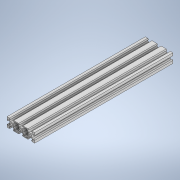
# Autodesk Inventor part: V-SLOT_2060
Saved by Autodesk Inventor 2021 (Build 250183000, 183)
## iProperties
Created: 2022-05-21
Part Number: V-SLOT_2060
Material: Genérico
Document SubType Name: Modeling
Designer: 79449
Density: 1 g/cm^3
Appearance: Valor por defecto
Author: 79449
Autodesk Inventor part; units mm, degrees
ref_plane "YZ Plane" through (0, 0, 0) normal (1, 0, 0) x (0, 1, 0)
ref_plane "XZ Plane" through (0, 0, 0) normal (0, 1, 0) x (-1, 0, 0)
ref_plane "XY Plane" through (0, 0, 0) normal (0, 0, 1) x (1, 0, 0)
sketch "Boceto1" plane through (0, 0, 0) normal (0, 0, 1) x (1, 0, 0)
  circle A0 centre (0, 0) radius 2.1
  line L0 (-2.8393, 3.9) -> (2.8393, 3.9)
  line L1 (3.9, 2.8393) -> (3.9, -2.8393)
  line L2 (2.8393, -3.9) -> (-2.8393, -3.9)
  line L3 (-3.9, -2.8393) -> (-3.9, 2.8393)
  line L4 (-3.9, 3.9) -> (3.9, -3.9) construction
  line L5 (3.9, 3.9) -> (-3.9, -3.9) construction
  line L6 (3.9, 3.9) -> (5.9093, 5.9093) construction
  line L7 (7, 5.9393) -> (3.9, 2.8393)
  line L8 (2.8393, 3.9) -> (5.5, 6.5607)
  line L9 (30, -10) -> (-30, -10) construction
  line L10 (-30, -10) -> (-30, 10) construction
  line L11 (-30, 10) -> (30, 10) construction
  line L12 (30, 10) -> (30, -10) construction
  line L13 (30, -10) -> (-30, 10) construction
  line L14 (-30, -10) -> (30, 10) construction
  line L15 (10, -10) -> (-10, -10) construction
  line L16 (-10, 10) -> (10, 10) construction
  line L17 (10, -10) -> (-10, 10) construction
  line L18 (-10, -10) -> (10, 10) construction
  line L19 (5.5, 6.5607) -> (5.5, 8.2)
  line L20 (7, 5.9393) -> (7, 8.2)
  line L21 (0, 10) -> (0, -10) construction
  line L22 (-3.9, 3.9) -> (-5.9093, 5.9093) construction
  line L23 (-7, 5.9393) -> (-3.9, 2.8393)
  line L24 (-2.8393, 3.9) -> (-5.5, 6.5607)
  line L25 (10, -10) -> (-10, 10) construction
  line L26 (-5.5, 6.5607) -> (-5.5, 8.2)
  line L27 (4.58, 10) -> (2.78, 8.2)
  line L28 (-4.58, 10) -> (-2.78, 8.2)
  line L29 (-7, 5.9393) -> (-7, 8.2)
  line L30 (-30, 0) -> (30, 0) construction
  line L31 (3.9, -3.9) -> (5.9093, -5.9093) construction
  line L32 (7, -5.9393) -> (3.9, -2.8393)
  line L33 (2.8393, -3.9) -> (5.5, -6.5607)
  line L34 (10, 10) -> (-10, -10) construction
  line L35 (-10, 10) -> (10, -10) construction
  line L36 (5.5, -6.5607) -> (5.5, -8.2)
  line L37 (7, -5.9393) -> (7, -8.2)
  line L38 (-5.5, -6.5607) -> (-5.5, -8.2)
  line L39 (-3.9, -3.9) -> (-5.9093, -5.9093) construction
  line L40 (-7, -5.9393) -> (-3.9, -2.8393)
  line L41 (-2.8393, -3.9) -> (-5.5, -6.5607)
  line L42 (10, 10) -> (-10, -10) construction
  line L43 (4.58, -10) -> (2.78, -8.2)
  line L44 (-4.58, -10) -> (-2.78, -8.2)
  line L45 (-7, -5.9393) -> (-7, -8.2)
  line L46 (-2.78, -8.2) -> (-5.5, -8.2)
  line L47 (5.5, -8.2) -> (2.78, -8.2)
  line L48 (7, -8.2) -> (10, -8.2)
  line L49 (-10, 8.2) -> (-7, 8.2)
  line L50 (-5.5, 8.2) -> (-2.78, 8.2)
  line L51 (2.78, 8.2) -> (5.5, 8.2)
  line L52 (7, 8.2) -> (10, 8.2)
  line L53 (-10, 8.2) -> (10, 8.2) construction
  line L54 (20, -10) -> (20, 10) construction
  line L55 (-10, -10) -> (-10, 10) construction
  line L56 (10, 10) -> (10, -10) construction
  line L57 (-4.58, 10) -> (-10, 10)
  line L58 (4.58, 10) -> (10, 10)
  line L59 (4.58, -10) -> (10, -10)
  line L60 (-4.58, -10) -> (-10, -10)
  circle A1 centre (20, 0) radius 2.1
  line L61 (22.8393, 3.9) -> (17.1607, 3.9)
  line L62 (16.1, 2.8393) -> (16.1, -2.8393)
  line L63 (17.1607, -3.9) -> (22.8393, -3.9)
  line L64 (23.9, -2.8393) -> (23.9, 2.8393)
  line L65 (23.9, 3.9) -> (16.1, -3.9) construction
  line L66 (16.1, 3.9) -> (23.9, -3.9) construction
  line L67 (16.1, 3.9) -> (14.0907, 5.9093) construction
  line L68 (13, 5.9393) -> (16.1, 2.8393)
  line L69 (17.1607, 3.9) -> (14.5, 6.5607)
  line L70 (-10, -10) -> (50, -10) construction
  line L71 (50, 10) -> (-10, 10) construction
  line L72 (-10, -10) -> (50, 10) construction
  line L73 (50, -10) -> (-10, 10) construction
  line L74 (10, -10) -> (30, -10) construction
  line L75 (30, 10) -> (10, 10) construction
  line L76 (10, -10) -> (30, 10) construction
  line L77 (30, -10) -> (10, 10) construction
  line L78 (14.5, 6.5607) -> (14.5, 8.2)
  line L79 (13, 5.9393) -> (13, 8.2)
  line L80 (20, 10) -> (20, -10) construction
  line L81 (25.5, 6.5607) -> (25.5, 8.2)
  line L82 (23.9, 3.9) -> (25.9093, 5.9093) construction
  line L83 (26.5607, 5.5) -> (23.9, 2.8393)
  line L84 (22.8393, 3.9) -> (25.5, 6.5607)
  line L85 (10, -10) -> (30, 10) construction
  line L86 (15.42, 10) -> (17.22, 8.2)
  line L87 (24.58, 10) -> (22.78, 8.2)
  line L88 (50, 0) -> (-10, 0) construction
  line L89 (16.1, -3.9) -> (14.0907, -5.9093) construction
  line L90 (30, 10) -> (10, -10) construction
  line L91 (13, -5.9393) -> (16.1, -2.8393)
  line L92 (17.1607, -3.9) -> (14.5, -6.5607)
  line L93 (14.5, -6.5607) -> (14.5, -8.2)
  line L94 (13, -5.9393) -> (13, -8.2)
  line L95 (15.42, -10) -> (17.22, -8.2)
  line L96 (27, -5.9393) -> (27, -8.2) construction
  line L97 (10, 10) -> (30, -10) construction
  line L98 (10, 10) -> (30, -10) construction
  line L99 (25.5, -6.5607) -> (25.5, -8.2)
  line L100 (26.5607, -5.5) -> (23.9, -2.8393)
  line L101 (23.9, -3.9) -> (25.9093, -5.9093) construction
  line L102 (22.8393, -3.9) -> (25.5, -6.5607)
  line L103 (24.58, -10) -> (22.78, -8.2)
  line L104 (22.78, -8.2) -> (25.5, -8.2)
  line L105 (27.1393, -8.2) -> (30, -8.2) construction
  line L106 (14.5, -8.2) -> (17.22, -8.2)
  line L107 (13, -8.2) -> (10, -8.2)
  line L108 (25.5, 8.2) -> (22.78, 8.2)
  line L109 (17.22, 8.2) -> (14.5, 8.2)
  line L110 (13, 8.2) -> (10, 8.2)
  line L111 (28.2, 8.2) -> (10, 8.2) construction
  line L112 (30, -10) -> (30, 10) construction
  line L113 (24.58, 10) -> (30, 10)
  line L114 (15.42, 10) -> (10, 10)
  line L115 (15.42, -10) -> (10, -10)
  line L116 (24.58, -10) -> (30, -10)
  circle A2 centre (-20, 0) radius 2.1
  line L117 (-17.1607, 3.9) -> (-22.8393, 3.9)
  line L118 (-23.9, 2.8393) -> (-23.9, -2.8393)
  line L119 (-22.8393, -3.9) -> (-17.1607, -3.9)
  line L120 (-16.1, -2.8393) -> (-16.1, 2.8393)
  line L121 (-16.1, 3.9) -> (-23.9, -3.9) construction
  line L122 (-23.9, 3.9) -> (-16.1, -3.9) construction
  line L123 (-23.9, 3.9) -> (-25.9093, 5.9093) construction
  line L124 (-26.5607, 5.5) -> (-23.9, 2.8393)
  line L125 (-22.8393, 3.9) -> (-25.5, 6.5607)
  line L126 (-50, -10) -> (10, -10) construction
  line L127 (10, 10) -> (-50, 10) construction
  line L128 (-50, -10) -> (10, 10) construction
  line L129 (10, -10) -> (-50, 10) construction
  line L130 (-30, -10) -> (-10, -10) construction
  line L131 (-10, 10) -> (-30, 10) construction
  line L132 (-30, -10) -> (-10, 10) construction
  line L133 (-10, -10) -> (-30, 10) construction
  line L134 (-25.5, 6.5607) -> (-25.5, 8.2)
  line L135 (-20, 10) -> (-20, -10) construction
  line L136 (-14.5, 6.5607) -> (-14.5, 8.2)
  line L137 (-16.1, 3.9) -> (-14.0907, 5.9093) construction
  line L138 (-13, 5.9393) -> (-16.1, 2.8393)
  line L139 (-17.1607, 3.9) -> (-14.5, 6.5607)
  line L140 (-30, -10) -> (-10, 10) construction
  line L141 (-24.58, 10) -> (-22.78, 8.2)
  line L142 (-15.42, 10) -> (-17.22, 8.2)
  line L143 (-13, 5.9393) -> (-13, 8.2)
  line L144 (10, 0) -> (-50, 0) construction
  line L145 (-23.9, -3.9) -> (-25.9093, -5.9093) construction
  line L146 (-10, 10) -> (-30, -10) construction
  line L147 (-26.5607, -5.5) -> (-23.9, -2.8393)
  line L148 (-22.8393, -3.9) -> (-25.5, -6.5607)
  line L149 (-25.5, -6.5607) -> (-25.5, -8.2)
  line L150 (-24.58, -10) -> (-22.78, -8.2)
  line L151 (-13, -5.9393) -> (-13, -8.2)
  line L152 (-30, 10) -> (-10, -10) construction
  line L153 (-30, 10) -> (-10, -10) construction
  line L154 (-14.5, -6.5607) -> (-14.5, -8.2)
  line L155 (-13, -5.9393) -> (-16.1, -2.8393)
  line L156 (-16.1, -3.9) -> (-14.0907, -5.9093) construction
  line L157 (-17.1607, -3.9) -> (-14.5, -6.5607)
  line L158 (-15.42, -10) -> (-17.22, -8.2)
  line L159 (-17.22, -8.2) -> (-14.5, -8.2)
  line L160 (-25.5, -8.2) -> (-22.78, -8.2)
  line L161 (-10, 8.2) -> (-13, 8.2)
  line L162 (-14.5, 8.2) -> (-17.22, 8.2)
  line L163 (-22.78, 8.2) -> (-25.5, 8.2)
  line L164 (-10, 8.2) -> (-25.5, 8.2) construction
  line L165 (-30, 10) -> (-30, -10) construction
  line L166 (-15.42, 10) -> (-10, 10)
  line L167 (-24.58, 10) -> (-30, 10)
  line L168 (-24.58, -10) -> (-30, -10)
  line L169 (-15.42, -10) -> (-10, -10)
  line L170 (-30, -10) -> (-50, -10) construction
  line L171 (-10, -10) -> (-70, -10) construction
  line L172 (-70, 10) -> (-10, 10) construction
  line L173 (-10, -10) -> (-70, 10) construction
  line L174 (-70, -10) -> (-10, 10) construction
  line L175 (-70, 0) -> (-10, 0) construction
  line L176 (-30, 10) -> (-50, -10) construction
  line L177 (-30, 10) -> (-50, -10) construction
  line L178 (-50, 10) -> (-30, -10) construction
  line L179 (-30, -10) -> (-50, 10) construction
  line L180 (-30, -10) -> (-50, 10) construction
  line L181 (-50, -10) -> (-30, 10) construction
  line L182 (-50, 8.2) -> (-30, 8.2) construction
  line L183 (-50, 10) -> (-30, 10) construction
  line L184 (-30, 10) -> (-30, 8.2)
  line L185 (-30, -8.2) -> (-30, -10)
  line L186 (30, -10) -> (30, -8.2)
  line L187 (30, 8.2) -> (30, 10)
  line L188 (28.2, -10) -> (28.2, -5.5) construction
  line L189 (28.2, -5.5) -> (28.2, -2.7333)
  line L190 (25.5, -6.5607) -> (26.5607, -5.5) construction
  line L191 (26.5607, -5.5) -> (28.2, -5.5)
  line L192 (28.2, -2.7333) -> (30, -4.5333)
  line L193 (30, -8.2) -> (30, -4.5333)
  line L194 (26.5607, 5.5) -> (23.9, 2.8393)
  line L195 (30, 10) -> (30, 8.2)
  line L196 (28.2, 5.5) -> (28.2, 2.7333)
  line L197 (26.5607, 5.5) -> (28.2, 5.5)
  line L198 (28.2, 2.7333) -> (30, 4.5333)
  line L199 (30, 8.2) -> (30, 4.5333)
  line L200 (-50, -10) -> (10, 10) construction
  line L201 (-28.2, -5.5) -> (-28.2, -2.7333)
  line L202 (-26.5607, -5.5) -> (-28.2, -5.5)
  line L203 (-28.2, -2.7333) -> (-30, -4.5333)
  line L204 (-30, -8.2) -> (-30, -4.5333)
  line L205 (-26.5607, 5.5) -> (-28.2, 5.5)
  line L206 (-28.2, 5.5) -> (-28.2, 2.7333)
  line L207 (-28.2, 2.7333) -> (-30, 4.5333)
  line L208 (-30, 8.2) -> (-30, 4.5333)
  line L209 (-10, -8.2) -> (-13, -8.2)
  line L210 (-10, -8.2) -> (-7, -8.2)
  dimension "d0" = 4.2
  dimension "d2" = 3.9
  dimension "d3" = 3.9
  dimension "d5" = 45
  dimension "d6" = 0.75
  dimension "d7" = 0.75
  dimension "d8" = 60
  dimension "d9" = 20
  dimension "d13" = 1.5
  dimension "d37" = 9.16
  dimension "d41" = 11
  dimension "d42" = 90
  dimension "d45" = 4.58
  dimension "d46" = 45
  dimension "d47" = 45
  dimension "d48" = 2.72
  dimension "d49" = 1.8
  dimension "d50" = 2.72
  dimension "d51" = 1.0607
  dimension "d53" = 10
  dimension "d54" = 20
  dimension "d55" = 3
  dimension "d56" = 1.6393
  dimension "d58" = 2.72
  dimension "d61" = 2.6607
  dimension "d62" = 3.4393
  dimension "d66" = 1.8
  dimension "d68" = 5.42
  dimension "d71" = 45
  dimension "d72" = 2.6607
  constraints: 422 end point, 153 symmetric about line, 28 point on line, 22 midpoint, 13 perpendicular, 8 parallel, 6 collinear, 5 horizontal, 3 centre point, 3 coincident, 1 vertical, 2 other
  measures "d0" diameter of A0
  measures "d2" distance from line of L1 point (0, 0)
  measures "d3" distance from line of L0 point (0, 0)
  measures "d5" angle of L6 L1
  measures "d6" distance between parallel lines of L6 L7
  measures "d7" distance between parallel lines of L6 L8
  measures "d8" distance of L10.end L11.end
  measures "d9" distance of L11.end L9.start
  measures "d13" distance between parallel lines of L20 L19
  measures "d37" distance of L28.start L27.start
  measures "d41" distance between parallel lines of L26 L19
  measures "d42" angle of L28 L27
  measures "d45" distance of L21.start L27.start
  measures "d46" angle of L28 L53
  measures "d47" angle of L27 L53
  measures "d48" distance of L27.end L19.end
  measures "d49" distance between parallel lines of L11 L53
  measures "d50" distance of L26.end L28.end
  measures "d51" horizontal distance of L2.end L3.start
  measures "d53" distance between parallel lines of L12 L54
  measures "d54" distance of L35.end L15.end
  measures "d55" distance of L37.end L48.end
  measures "d56" distance of L99.start L104.end
  measures "d58" distance of L104.start L104.end
  measures "d61" horizontal distance of L63.start L92.end
  measures "d62" distance from line of L74 L99.start
  measures "d66" distance between parallel lines of L188 L112
  measures "d68" distance of L74.end L103.start
  measures "d71" angle of L189 L192
  measures "d72" horizontal distance of L100.start L64.start
extrude "Extrusión1" add sketch "Boceto1" along normal blind 300
